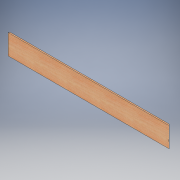
# Autodesk Inventor part: SkinnySideLengthPower
Saved by Autodesk Inventor 2016 (Build 200138000, 138)
## iProperties
Created: 2016-02-11
Part Number: SkinnySideLengthPower
Material: Wood (Birch)
Document SubType Name: Modeling
Designer: ron
Density: 0.55 g/cm^3
Appearance: Birch - Natural Polished
Mass: 1723.3 g
Surface Area: 4352.45 cm^2
Volume: 3133.27 cm^3
Author: ron
Autodesk Inventor part; units mm, degrees
ref_plane "YZ Plane" through (0, 0, 0) normal (1, 0, 0) x (0, 1, 0)
ref_plane "XZ Plane" through (0, 0, 0) normal (0, 1, 0) x (-1, 0, 0)
sketch "Sketch1" plane through (0, 0, 0) normal (1, 0, 0) x (0, 1, 0)
  line L0 (0, 0) -> (155.1, 0)
  line L1 (155.1, 0) -> (155.1, -10)
  line L2 (0, -20) -> (0, 0)
  line L3 (155.1, -10) -> (101.6, -10)
  line L4 (101.6, -10) -> (101.6, -20)
  line L5 (101.6, -20) -> (0, -20)
  dimension "d3" = 53.5
  dimension "d4" = 155.1
  dimension "d5" = 10
  dimension "d6" = 10
  dimension "d7" = 20
  dimension "d18" = 101.6
  constraints: 12 end point, 3 horizontal, 2 parallel, 1 perpendicular
  measures "d3" distance of L1.end L3.end
  measures "d4" distance between parallel lines of L1 L2
  measures "d5" distance between parallel lines of L3 L5
  measures "d6" distance between parallel lines of L0 L3
  measures "d7" vertical distance of L4.end L0.end
  measures "d18" distance of L4.end L2.start
extrude "Extrusion1" add sketch "Sketch1" along normal blind 1238.8342
chamfer "Chamfer1" distance 19.812 angle 45 1 edges at (1238.8342, 50.8, -20)
chamfer "Chamfer2" distance 19.812 angle 45 1 edges at (0, 50.8, -20)
ref_plane "Work Plane2" through (1183.1012, 38.0112, -55.921) normal (-0.7071, 0, -0.7071) x (0, 1, 0)
sketch "Sketch3" plane through (1183.1012, 38.0112, -55.921) normal (-0.7071, 0, -0.7071) x (0, 1, 0)
  line L0 (117.0888, 0) -> (14.7014, 0)
  point P0 (-38.0112, -876.121)
  dimension "d21" = 102.3874
  constraints: 2 end point
  measures "d21" distance of L0.start L0.end
hole "Hole1" at (1183.1012, 52.7126, -55.921) direction (0.7071, 0, 0.7071) diameter 12.7 depth 127 tip angle 118
body "Solid1"
